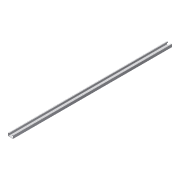
# Autodesk Inventor part: Unistrut 4ft
Saved by Autodesk Inventor 2014 (Build 180170000, 170)
## iProperties
Created: 2014-07-12
Part Number: Unistrut 4ft
Material: Generic
Document SubType Name: Modeling
Designer: Owner
Density: 1 g/cm^3
Appearance: Aluminum - Polished
Author: Owner
Autodesk Inventor part; units mm, degrees
ref_plane "YZ Plane" through (0, 0, 0) normal (1, 0, 0) x (0, 1, 0)
ref_plane "XZ Plane" through (0, 0, 0) normal (0, 1, 0) x (-1, 0, 0)
ref_plane "XY Plane" through (0, 0, 0) normal (0, 0, 1) x (1, 0, 0)
sketch "Sketch1" plane through (0, 0, 0) normal (0, 0, 1) x (1, 0, 0)
  line L0 (0, 0) -> (41.275, 0) construction
  line L1 (41.275, 0) -> (41.275, 22.225) construction
  line L2 (41.275, 22.225) -> (0, 22.225) construction
  line L3 (0, 22.225) -> (0, 0) construction
  line L4 (3.175, 0) -> (38.1, 0)
  line L5 (41.275, 19.05) -> (41.275, 3.175)
  line L6 (38.1, 22.225) -> (34.925, 22.225)
  line L7 (31.75, 19.05) -> (31.75, 15.4623)
  line L8 (0, 3.175) -> (0, 19.05)
  line L9 (3.175, 22.225) -> (6.35, 22.225)
  line L10 (9.525, 19.05) -> (9.525, 15.4622)
  line L11 (1.5748, 17.4752) -> (1.5748, 4.7498)
  line L12 (4.7498, 20.6502) -> (4.7752, 20.6502)
  line L13 (36.5252, 20.6502) -> (36.4998, 20.6502)
  line L14 (39.7002, 4.7498) -> (39.7002, 17.4752)
  line L15 (33.3248, 17.4752) -> (33.3248, 15.4623)
  line L16 (7.9502, 17.4752) -> (7.9502, 15.4622)
  line L17 (4.7498, 1.5748) -> (36.5252, 1.5748)
  arc A0 (3.175, 22.225) -> (0, 19.05) centre (3.175, 19.05) ccw
  arc A1 (9.525, 19.05) -> (6.35, 22.225) centre (6.35, 19.05) ccw
  arc A2 (7.9502, 17.4752) -> (4.7752, 20.6502) centre (4.7752, 17.4752) ccw
  arc A3 (4.7498, 20.6502) -> (1.5748, 17.4752) centre (4.7498, 17.4752) ccw
  arc A4 (34.925, 22.225) -> (31.75, 19.05) centre (34.925, 19.05) ccw
  arc A5 (41.275, 19.05) -> (38.1, 22.225) centre (38.1, 19.05) ccw
  arc A6 (39.7002, 17.4752) -> (36.5252, 20.6502) centre (36.5252, 17.4752) ccw
  arc A7 (36.4998, 20.6502) -> (33.3248, 17.4752) centre (36.4998, 17.4752) ccw
  arc A8 (36.5252, 1.5748) -> (39.7002, 4.7498) centre (36.5252, 4.7498) ccw
  arc A9 (1.5748, 4.7498) -> (4.7498, 1.5748) centre (4.7498, 4.7498) ccw
  arc A10 (0, 3.175) -> (3.175, 0) centre (3.175, 3.175) ccw
  arc A11 (38.1, 0) -> (41.275, 3.175) centre (38.1, 3.175) ccw
  line L18 (8.3312, 15.0812) -> (9.144, 15.0812)
  line L19 (32.131, 15.0813) -> (32.9438, 15.0813)
  arc A12 (7.9502, 15.4622) -> (8.3312, 15.0812) centre (8.3312, 15.4622) ccw
  arc A13 (9.144, 15.0812) -> (9.525, 15.4622) centre (9.144, 15.4622) ccw
  arc A14 (31.75, 15.4623) -> (32.131, 15.0813) centre (32.131, 15.4623) ccw
  arc A15 (32.9438, 15.0813) -> (33.3248, 15.4623) centre (32.9438, 15.4623) ccw
  point P0 (31.75, 22.225)
  point P1 (31.75, 15.0813)
  point P2 (9.525, 22.225)
  point P3 (9.525, 15.0812)
  point P4 (1.5748, 1.5748)
  point P5 (1.5748, 20.6502)
  point P6 (7.9502, 20.6502)
  point P7 (33.3248, 20.6502)
  point P8 (39.7002, 1.5748)
  point P9 (33.3248, 15.0813)
  point P10 (7.9502, 15.0812)
  dimension "d7" = 41.275
  dimension "d8" = 22.225
  dimension "d9" = 9.525
  dimension "d10" = 7.1437
  dimension "d11" = 9.525
  dimension "d12" = 7.1437
  dimension "d13" = 1.5748
  dimension "d14" = 1.5748
  dimension "d15" = 1.5748
  dimension "d18" = 1.5748
  dimension "d19" = 1.5748
  dimension "d20" = 1.5748
  dimension "d21" = 1.5748
  dimension "d22" = 1.5748
  dimension "d23" = 1.5748
  dimension "d24" = 1.5748
  dimension "d25" = 1.5748
  dimension "d26" = 5.569
  dimension "d27" = 5.569
  dimension "d28" = 3.175
  dimension "d29" = 3.175
  dimension "d30" = 0.381
  constraints: 40 end point, 32 point on circle, 32 point on line, 32 tangent, 16 centre point, 13 equal radius, 8 parallel, 4 perpendicular, 1 coincident, 1 collinear, 1 horizontal, 1 other
  measures "d7" distance of L1.end L2.end
  measures "d8" distance of L0.end L1.end
  measures "d9" distance of L1.end point (31.75, 22.225)
  measures "d10" distance of point (31.75, 22.225) point (31.75, 15.081)
  measures "d11" distance of L2.end point (9.525, 22.225)
  measures "d12" distance of point (9.525, 22.225) point (9.525, 15.081)
  measures "d13" distance between parallel lines of L3 L11
  measures "d14" distance between parallel lines of L9 L12
  measures "d15" distance between parallel lines of L2 L13
  measures "d18" horizontal distance of L2.end point (1.575, 20.65)
  measures "d19" horizontal distance of L2.end point (1.575, 20.65)
  measures "d20" distance between parallel lines of L10 L16
  measures "d21" distance between parallel lines of L15 L7
  measures "d22" distance between parallel lines of L1 L14
  measures "d23" horizontal distance of point (9.525, 22.225) point (7.95, 20.65)
  measures "d24" distance from line of L0 point (1.575, 1.575)
  measures "d25" distance from line of L0 point (39.7, 1.575)
  measures "d26" distance of point (7.95, 20.65) point (7.95, 15.081)
  measures "d27" distance of point (33.325, 20.65) point (33.325, 15.081)
  measures "d28" radius of A0
  measures "d29" radius of A10
  measures "d30" radius of A12
extrude "Extrusion2" add sketch "Sketch1" against normal blind 1219.2
sketch "Sketch5" plane through (3.175, 0, 0) normal (0, -1, 0) x (1, 0, 0)
  line L0 (34.925, 0) -> (34.925, -1219.2) projected
  line L1 (0, -1219.2) -> (34.925, -1219.2) construction
  line L2 (0, 0) -> (34.925, 0) construction
  line L3 (17.4625, 0) -> (17.4625, -1219.2) construction
  line L4 (17.4625, -1219.2) -> (17.4625, -1200.15) construction
  line L5 (17.4625, -1200.15) -> (17.4625, -1185.8625) construction
  line L6 (24.6062, -1200.15) -> (24.6062, -1185.8625)
  line L7 (10.3187, -1185.8625) -> (10.3187, -1200.15)
  arc A0 (10.3187, -1200.15) -> (24.6062, -1200.15) centre (17.4625, -1200.15) ccw
  arc A1 (24.6062, -1185.8625) -> (10.3187, -1185.8625) centre (17.4625, -1185.8625) ccw
  line L8 (17.4625, -1149.35) -> (17.4625, -1135.0625) construction
  line L9 (24.6062, -1149.35) -> (24.6062, -1135.0625)
  line L10 (10.3187, -1135.0625) -> (10.3187, -1149.35)
  arc A2 (10.3187, -1149.35) -> (24.6062, -1149.35) centre (17.4625, -1149.35) ccw
  arc A3 (24.6062, -1135.0625) -> (10.3187, -1135.0625) centre (17.4625, -1135.0625) ccw
  line L11 (17.4625, -1098.55) -> (17.4625, -1084.2625) construction
  line L12 (24.6062, -1098.55) -> (24.6062, -1084.2625)
  line L13 (10.3187, -1084.2625) -> (10.3187, -1098.55)
  arc A4 (10.3187, -1098.55) -> (24.6062, -1098.55) centre (17.4625, -1098.55) ccw
  arc A5 (24.6062, -1084.2625) -> (10.3187, -1084.2625) centre (17.4625, -1084.2625) ccw
  line L14 (17.4625, -1047.75) -> (17.4625, -1033.4625) construction
  line L15 (24.6062, -1047.75) -> (24.6062, -1033.4625)
  line L16 (10.3187, -1033.4625) -> (10.3187, -1047.75)
  arc A6 (10.3187, -1047.75) -> (24.6062, -1047.75) centre (17.4625, -1047.75) ccw
  arc A7 (24.6062, -1033.4625) -> (10.3187, -1033.4625) centre (17.4625, -1033.4625) ccw
  line L17 (17.4625, -996.95) -> (17.4625, -982.6625) construction
  line L18 (24.6062, -996.95) -> (24.6062, -982.6625)
  line L19 (10.3187, -982.6625) -> (10.3187, -996.95)
  arc A8 (10.3187, -996.95) -> (24.6062, -996.95) centre (17.4625, -996.95) ccw
  arc A9 (24.6062, -982.6625) -> (10.3187, -982.6625) centre (17.4625, -982.6625) ccw
  line L20 (17.4625, -946.15) -> (17.4625, -931.8625) construction
  line L21 (24.6062, -946.15) -> (24.6062, -931.8625)
  line L22 (10.3187, -931.8625) -> (10.3187, -946.15)
  arc A10 (10.3187, -946.15) -> (24.6062, -946.15) centre (17.4625, -946.15) ccw
  arc A11 (24.6062, -931.8625) -> (10.3187, -931.8625) centre (17.4625, -931.8625) ccw
  line L23 (17.4625, -895.35) -> (17.4625, -881.0625) construction
  line L24 (24.6062, -895.35) -> (24.6062, -881.0625)
  line L25 (10.3187, -881.0625) -> (10.3187, -895.35)
  arc A12 (10.3187, -895.35) -> (24.6062, -895.35) centre (17.4625, -895.35) ccw
  arc A13 (24.6062, -881.0625) -> (10.3187, -881.0625) centre (17.4625, -881.0625) ccw
  line L26 (17.4625, -844.55) -> (17.4625, -830.2625) construction
  line L27 (24.6062, -844.55) -> (24.6062, -830.2625)
  line L28 (10.3187, -830.2625) -> (10.3187, -844.55)
  arc A14 (10.3187, -844.55) -> (24.6062, -844.55) centre (17.4625, -844.55) ccw
  arc A15 (24.6062, -830.2625) -> (10.3187, -830.2625) centre (17.4625, -830.2625) ccw
  line L29 (17.4625, -793.75) -> (17.4625, -779.4625) construction
  line L30 (24.6062, -793.75) -> (24.6062, -779.4625)
  line L31 (10.3187, -779.4625) -> (10.3187, -793.75)
  arc A16 (10.3187, -793.75) -> (24.6062, -793.75) centre (17.4625, -793.75) ccw
  arc A17 (24.6062, -779.4625) -> (10.3187, -779.4625) centre (17.4625, -779.4625) ccw
  line L32 (17.4625, -742.95) -> (17.4625, -728.6625) construction
  line L33 (24.6062, -742.95) -> (24.6062, -728.6625)
  line L34 (10.3187, -728.6625) -> (10.3187, -742.95)
  arc A18 (10.3187, -742.95) -> (24.6062, -742.95) centre (17.4625, -742.95) ccw
  arc A19 (24.6062, -728.6625) -> (10.3187, -728.6625) centre (17.4625, -728.6625) ccw
  line L35 (17.4625, -692.15) -> (17.4625, -677.8625) construction
  line L36 (24.6062, -692.15) -> (24.6062, -677.8625)
  line L37 (10.3187, -677.8625) -> (10.3187, -692.15)
  arc A20 (10.3187, -692.15) -> (24.6062, -692.15) centre (17.4625, -692.15) ccw
  arc A21 (24.6062, -677.8625) -> (10.3187, -677.8625) centre (17.4625, -677.8625) ccw
  line L38 (17.4625, -641.35) -> (17.4625, -627.0625) construction
  line L39 (24.6062, -641.35) -> (24.6062, -627.0625)
  line L40 (10.3187, -627.0625) -> (10.3187, -641.35)
  arc A22 (10.3187, -641.35) -> (24.6062, -641.35) centre (17.4625, -641.35) ccw
  arc A23 (24.6062, -627.0625) -> (10.3187, -627.0625) centre (17.4625, -627.0625) ccw
  line L41 (17.4625, -590.55) -> (17.4625, -576.2625) construction
  line L42 (24.6062, -590.55) -> (24.6062, -576.2625)
  line L43 (10.3187, -576.2625) -> (10.3187, -590.55)
  arc A24 (10.3187, -590.55) -> (24.6062, -590.55) centre (17.4625, -590.55) ccw
  arc A25 (24.6062, -576.2625) -> (10.3187, -576.2625) centre (17.4625, -576.2625) ccw
  line L44 (17.4625, -539.75) -> (17.4625, -525.4625) construction
  line L45 (24.6062, -539.75) -> (24.6062, -525.4625)
  line L46 (10.3187, -525.4625) -> (10.3187, -539.75)
  arc A26 (10.3187, -539.75) -> (24.6062, -539.75) centre (17.4625, -539.75) ccw
  arc A27 (24.6062, -525.4625) -> (10.3187, -525.4625) centre (17.4625, -525.4625) ccw
  line L47 (17.4625, -488.95) -> (17.4625, -474.6625) construction
  line L48 (24.6062, -488.95) -> (24.6062, -474.6625)
  line L49 (10.3187, -474.6625) -> (10.3187, -488.95)
  arc A28 (10.3187, -488.95) -> (24.6062, -488.95) centre (17.4625, -488.95) ccw
  arc A29 (24.6062, -474.6625) -> (10.3187, -474.6625) centre (17.4625, -474.6625) ccw
  line L50 (17.4625, -438.15) -> (17.4625, -423.8625) construction
  line L51 (24.6062, -438.15) -> (24.6062, -423.8625)
  line L52 (10.3187, -423.8625) -> (10.3187, -438.15)
  arc A30 (10.3187, -438.15) -> (24.6062, -438.15) centre (17.4625, -438.15) ccw
  arc A31 (24.6062, -423.8625) -> (10.3187, -423.8625) centre (17.4625, -423.8625) ccw
  line L53 (17.4625, -387.35) -> (17.4625, -373.0625) construction
  line L54 (24.6062, -387.35) -> (24.6062, -373.0625)
  line L55 (10.3187, -373.0625) -> (10.3187, -387.35)
  arc A32 (10.3187, -387.35) -> (24.6062, -387.35) centre (17.4625, -387.35) ccw
  arc A33 (24.6062, -373.0625) -> (10.3187, -373.0625) centre (17.4625, -373.0625) ccw
  line L56 (17.4625, -336.55) -> (17.4625, -322.2625) construction
  line L57 (24.6062, -336.55) -> (24.6062, -322.2625)
  line L58 (10.3187, -322.2625) -> (10.3187, -336.55)
  arc A34 (10.3187, -336.55) -> (24.6062, -336.55) centre (17.4625, -336.55) ccw
  arc A35 (24.6062, -322.2625) -> (10.3187, -322.2625) centre (17.4625, -322.2625) ccw
  line L59 (17.4625, -285.75) -> (17.4625, -271.4625) construction
  line L60 (24.6062, -285.75) -> (24.6062, -271.4625)
  line L61 (10.3187, -271.4625) -> (10.3187, -285.75)
  arc A36 (10.3187, -285.75) -> (24.6062, -285.75) centre (17.4625, -285.75) ccw
  arc A37 (24.6062, -271.4625) -> (10.3187, -271.4625) centre (17.4625, -271.4625) ccw
  line L62 (17.4625, -234.95) -> (17.4625, -220.6625) construction
  line L63 (24.6062, -234.95) -> (24.6062, -220.6625)
  line L64 (10.3187, -220.6625) -> (10.3187, -234.95)
  arc A38 (10.3187, -234.95) -> (24.6062, -234.95) centre (17.4625, -234.95) ccw
  arc A39 (24.6062, -220.6625) -> (10.3187, -220.6625) centre (17.4625, -220.6625) ccw
  line L65 (17.4625, -184.15) -> (17.4625, -169.8625) construction
  line L66 (24.6062, -184.15) -> (24.6062, -169.8625)
  line L67 (10.3187, -169.8625) -> (10.3187, -184.15)
  arc A40 (10.3187, -184.15) -> (24.6062, -184.15) centre (17.4625, -184.15) ccw
  arc A41 (24.6062, -169.8625) -> (10.3187, -169.8625) centre (17.4625, -169.8625) ccw
  line L68 (17.4625, -133.35) -> (17.4625, -119.0625) construction
  line L69 (24.6062, -133.35) -> (24.6062, -119.0625)
  line L70 (10.3187, -119.0625) -> (10.3187, -133.35)
  arc A42 (10.3187, -133.35) -> (24.6062, -133.35) centre (17.4625, -133.35) ccw
  arc A43 (24.6062, -119.0625) -> (10.3187, -119.0625) centre (17.4625, -119.0625) ccw
  line L71 (17.4625, -82.55) -> (17.4625, -68.2625) construction
  line L72 (24.6062, -82.55) -> (24.6062, -68.2625)
  line L73 (10.3187, -68.2625) -> (10.3187, -82.55)
  arc A44 (10.3187, -82.55) -> (24.6062, -82.55) centre (17.4625, -82.55) ccw
  arc A45 (24.6062, -68.2625) -> (10.3187, -68.2625) centre (17.4625, -68.2625) ccw
  line L74 (17.4625, -31.75) -> (17.4625, -17.4625) construction
  line L75 (24.6062, -31.75) -> (24.6062, -17.4625)
  line L76 (10.3187, -17.4625) -> (10.3187, -31.75)
  arc A46 (10.3187, -31.75) -> (24.6062, -31.75) centre (17.4625, -31.75) ccw
  arc A47 (24.6062, -17.4625) -> (10.3187, -17.4625) centre (17.4625, -17.4625) ccw
  point P0 (17.4625, -1193.0062)
  point P1 (17.4625, -1142.2062)
  point P2 (17.4625, -1091.4062)
  point P3 (17.4625, -1040.6063)
  point P4 (17.4625, -989.8063)
  point P5 (17.4625, -939.0062)
  point P6 (17.4625, -888.2062)
  point P7 (17.4625, -837.4062)
  point P8 (17.4625, -786.6062)
  point P9 (17.4625, -735.8062)
  point P10 (17.4625, -685.0063)
  point P11 (17.4625, -634.2062)
  point P12 (17.4625, -583.4062)
  point P13 (17.4625, -532.6062)
  point P14 (17.4625, -481.8062)
  point P15 (17.4625, -431.0062)
  point P16 (17.4625, -380.2062)
  point P17 (17.4625, -329.4062)
  point P18 (17.4625, -278.6062)
  point P19 (17.4625, -227.8063)
  point P20 (17.4625, -177.0063)
  point P21 (17.4625, -126.2062)
  point P22 (17.4625, -75.4062)
  point P23 (17.4625, -24.6062)
  dimension "d40" = 19.05
  dimension "d41" = 14.2875
  dimension "d42" = 14.2875
  dimension "d45" = 50.8
  constraints: 200 end point, 96 point on circle, 48 centre point, 4 tangent, 3 midpoint, 2 perpendicular, 2 point on line, 1 parallel, 1 vertical, 276 other
  measures "d40" distance of L3.end L4.end
  measures "d41" distance of L4.end L5.end
  measures "d42" diameter of A1
  measures "d45" distance of L6.start L9.start
extrude "Extrusion4" cut sketch "Sketch5" against normal blind 1.5773
equation "\"d14\" = d13"
equation "\"d15\" = d13"
equation "\"d20\" = d13"
equation "\"d21\" = d13"
equation "\"d22\" = d13"
equation "\"d24\" = d13"
equation "\"d25\" = d13"
body "Solid2"
